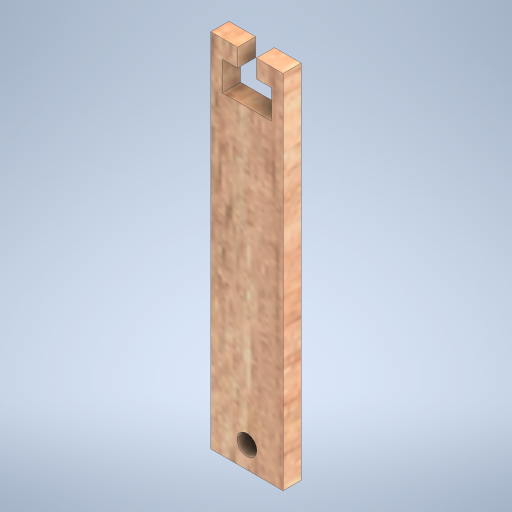
# Autodesk Inventor part: Leg1
Saved by Autodesk Inventor 2023 (Build 270158000, 158)
## iProperties
Created: 2023-11-27
Part Number: Leg1
Material: Wood (Birch)
Document SubType Name: Modeling
Designer: Mustapha
Mass: 10.6293 g
Surface Area: 101.444 cm^2
Volume: 19.326 cm^3
Density: 0.55 g/cm^3
Appearance: Birch - Natural Polished
Author: Mustapha
Autodesk Inventor part; units mm, degrees
ref_plane "YZ Plane" through (0, 0, 0) normal (1, 0, 0) x (0, 1, 0)
ref_plane "XZ Plane" through (0, 0, 0) normal (0, 1, 0) x (-1, 0, 0)
ref_plane "XY Plane" through (0, 0, 0) normal (0, 0, 1) x (1, 0, 0)
sketch "Sketch1" plane through (0, 0, 0) normal (0, 0, 1) x (1, 0, 0)
  line L0 (0, 0) -> (20, 0)
  line L1 (20, 0) -> (20, 100)
  line L2 (20, 100) -> (0, 100)
  line L3 (0, 100) -> (0, 0)
  dimension "d0" = 20
  dimension "d1" = 100
  constraints: 8 end point, 2 parallel, 1 horizontal, 1 perpendicular
  measures "d0" distance between parallel lines of L1 L3
  measures "d1" distance of L2.end L0.start
extrude "Extrusion1" add sketch "Sketch1" along normal blind 5
sketch "Sketch2" plane through (0, 0, 5) normal (0, 0, 1) x (1, 0, 0)
  line L0 (20, 100) -> (0, 100) projected
  line L1 (7.4, 100) -> (7.4, 95)
  line L2 (7.4, 95) -> (3.2, 95)
  line L3 (3.2, 95) -> (3.2, 87)
  line L4 (3.2, 87) -> (10, 87)
  line L5 (10, 87) -> (10, 204.0933)
  line L6 (7.4, 100) -> (10, 100)
  line L7 (20, 0) -> (20, 100) projected
  line L8 (0, 100) -> (20, 100)
  line L9 (12.6, 100) -> (12.6, 95)
  line L10 (12.6, 95) -> (16.8, 95)
  line L11 (16.8, 95) -> (16.8, 87)
  line L12 (16.8, 87) -> (10, 87)
  line L13 (12.6, 100) -> (10, 100)
  circle A0 centre (10, 6) radius 2.75
  line L14 (0, 0) -> (20, 0) projected
  dimension "d4" = 2.6
  dimension "d5" = 8
  dimension "d6" = 5
  dimension "d7" = 10
  dimension "d8" = 4.2
  dimension "d11" = 5.5
  dimension "d12" = 10
  dimension "d13" = 6
  constraints: 24 end point, 6 symmetric about line, 4 perpendicular, 3 point on line, 2 midpoint, 1 centre point, 1 vertical
  measures "d4" distance between parallel lines of L5 L1
  measures "d5" distance between parallel lines of L4 L2
  measures "d6" distance between parallel lines of L0 L2
  measures "d7" distance between parallel lines of L7 L5
  measures "d8" distance between parallel lines of L1 L3
  measures "d11" diameter of A0
  measures "d12" distance from line of L7 A0.centre
  measures "d13" distance from line of L14 A0.centre
extrude "Extrusion2" cut sketch "Sketch2" against normal blind 5
body "Solid1"
